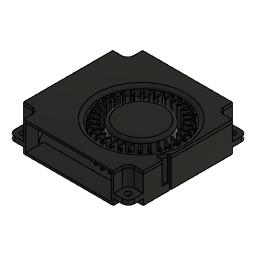
Fan centrifugal 40x40x10 v9 (Autodesk Fusion 360 design; units mm, degrees)
Autodesk Fusion 360 part; units mm, degrees
note: some values were not read from the file. Set by a fixed rule: which face or edge a step refers to; which sketch regions a step uses.
(part 1 of 2)
sketch "Sketch1" plane through (0, 0, 0) normal (0, 0, 1) x (1, 0, 0) in component "base"
  line L0 (18, 19.9) -> (-18, 19.9)
  line L1 (-18, -19.9) -> (18, -19.9)
  arc A0 (-20, -17.9) -> (-18, -19.9) centre (-18, -17.9) ccw
  line L2 (-15, -19.9) -> (-15, -16.9)
  line L3 (15, -16.9) -> (15, -19.9)
  line L4 (-20, 17.9) -> (-20, -17.9)
  arc A1 (-18, 19.9) -> (-20, 17.9) centre (-18, 17.9) ccw
  line L5 (-17, -14.9) -> (-20, -14.9)
  arc A2 (18.3387, -8.5746) -> (17.9789, -8) centre (18.3387, -8.1746) cw
  arc A3 (20, 17.9) -> (18, 19.9) centre (18, 17.9) ccw
  arc A4 (17, -14.9) -> (15, -16.9) centre (17, -16.9) ccw
  line L6 (17.9789, -8) -> (19.0465, -5.8)
  line L7 (19.4063, -5.5746) -> (20, -5.5746)
  arc A5 (19.0465, -5.8) -> (19.4063, -5.5746) centre (19.4063, -5.9746) cw
  line L8 (20, -17.9) -> (20, 17.9)
  circle A6 centre (17.5, -17.5) radius 1
  circle A7 centre (17.5, 17.5) radius 1
  line L9 (19.5, -5.5746) -> (19.5, -8.5746)
  line L10 (20, -14.9) -> (17, -14.9)
  circle A8 centre (-17.5, -17.5) radius 1
  arc A9 (-15, -16.9) -> (-17, -14.9) centre (-17, -16.9) ccw
  circle A10 centre (-17.5, 17.5) radius 1
  arc A11 (18, -19.9) -> (20, -17.9) centre (18, -17.9) ccw
  line L11 (20, -8.5746) -> (18.3387, -8.5746)
  line L12 (18, 17.9) -> (-18, -17.9) construction
  line L13 (-18, 17.9) -> (18, -17.9) construction
  line L14 (0, 0) -> (0, 8.903) construction
  line L15 (17.9789, -8) -> (17.7, -8.5746) construction
  line L16 (18.3387, -8.5746) -> (17.7, -8.5746) construction
  line L17 (0, 0) -> (8.2242, 0) construction
  line L18 (-15, 19.9) -> (-15, 16.9)
  arc A12 (-17, 14.9) -> (-15, 16.9) centre (-17, 16.9) ccw
  line L19 (-17, 14.9) -> (-20, 14.9)
  line L20 (15, 19.9) -> (15, 16.9)
  arc A13 (15, 16.9) -> (17, 14.9) centre (17, 16.9) ccw
  line L21 (17, 14.9) -> (20, 14.9)
  line L22 (14, -19.9) -> (14, -10.4)
  line L23 (-14, -19.9) -> (-14, -15.9)
  line L24 (19.5, 8.2159) -> (19.5, -2.135) construction
  line L25 (-2.9229, 19.25) -> (4.8128, 19.25) construction
  arc A14 (14, -10.4) -> (19.5, 1.2082) centre (4.5, 1.2082) ccw
  arc A15 (19.5, 1.2082) -> (1.4582, 19.25) centre (1.4582, 1.2082) ccw
  arc A16 (1.4582, 19.25) -> (-19.5, -1.7082) centre (1.4582, -1.7082) ccw
  line L26 (-19.5, 5.9603) -> (-19.5, -4.1012) construction
  arc A17 (-19.5, -1.7082) -> (-14, -15.9) centre (1.5598, -1.7082) ccw
  line L27 (19.5, -6.0746) -> (20, -6.0746)
  circle A18 centre (0, 0) radius 12.5
  circle A19 centre (4.5, -0.1) radius 3
  line L28 (4.5, -0.1) -> (18.5127, -6.9) construction
  line L29 (18.1641, -8.5345) -> (12.3384, -5.7074)
  line L30 (19.5, -5.5746) -> (13.7556, -2.787)
  line L31 (13.92, -2.4482) -> (12.1736, -6.0469)
  arc A20 (10.8374, -6.51) -> (12.1736, -6.0469) centre (11.274, -5.6103) ccw
  line L32 (10.8374, -6.51) -> (7.6886, -4.9819)
  arc A21 (7.2255, -3.6457) -> (7.6886, -4.9819) centre (8.1251, -4.0822) ccw
  line L33 (7.2255, -3.6457) -> (8.9718, -0.047)
  arc A22 (10.3081, 0.4161) -> (8.9718, -0.047) centre (9.8715, -0.4836) ccw
  line L34 (10.3081, 0.4161) -> (13.4569, -1.112)
  arc A23 (13.92, -2.4482) -> (13.4569, -1.112) centre (13.0203, -2.0116) ccw
  dimension "d2" = 40
  dimension "d3" = 39.8
  dimension "d10" = 2
  dimension "d12" = 2
  dimension "d13" = 5
  dimension "d18" = 3
  dimension "d21" = 35
  dimension "d22" = 35
  dimension "d23" = 0.5
  dimension "d26" = 2.3
  dimension "d27" = 5
  dimension "d28" = 5
  dimension "d29" = 2
  dimension "d30" = 0.4
  dimension "d31" = 9.5
  dimension "d32" = 28
  dimension "d33" = 0.5
  dimension "d34" = 0.65
  dimension "d35" = 0.5
  dimension "d36" = 4
  dimension "d37" = 15
  dimension "d38" = 0.5
  dimension "d97" = 25
  dimension "d98" = 6
  dimension "d99" = 15.5
  dimension "d100" = 20
  dimension "d101" = 8
  dimension "d102" = 1
  dimension "d103" = 6
  dimension "d104" = 9.5
  dimension "d105" = 5.5
  constraint coincident L9.start L7
  constraint tangent L0 A1
  constraint tangent L4 A1
  constraint tangent A3 L8
  constraint tangent L0 A3
  constraint tangent L5 A9
  constraint tangent A0 L4
  constraint tangent L8 A11
  constraint tangent A4 L10
  constraint tangent A2 L11
  constraint tangent A2 L6
  constraint tangent L7 A5
  constraint tangent L6 A5
  constraint coincident A3.centre L12.start
  constraint coincident A0.centre L12.end
  constraint coincident A1.centre L13.start
  constraint coincident A11.centre L13.end
  constraint midpoint L12 L14.start
  constraint equal A7 A10
  constraint equal A6 A7
  constraint equal A6 A8
  constraint equal A1 A3
  constraint equal A3 A11
  constraint equal A0 A11
  constraint equal A4 A9
  constraint vertical L4
  constraint vertical L8
  constraint horizontal L0
  constraint horizontal L1
  constraint tangent L1 A0
  constraint tangent L1 A11
  constraint coincident L9.end L11
  constraint horizontal L11
  constraint vertical L9
  constraint horizontal L7
  constraint horizontal L10
  constraint vertical L3
  constraint vertical L2
  constraint horizontal L5
  constraint tangent L2 A9
  constraint collinear L5 L10
  constraint coincident L14.start L17.start
  constraint parallel L6 L15
  constraint parallel L11 L16
  constraint equal A2 A5
  constraint tangent L3 A4
  constraint vertical L14
  constraint horizontal L17
  constraint symmetric A6.centre A7.centre L17
  constraint symmetric A8.centre A10.centre L17
  constraint symmetric A6.centre A8.centre L14
  constraint coincident L10.start L8
  constraint coincident L3.start A4.end
  constraint coincident L3.end L1
  constraint coincident L5.end L4
  constraint coincident L2.start L1
  constraint coincident L2.end A9.start
  constraint symmetric L3.end L2.start L14
  constraint coincident L0 L18.start
  constraint tangent L18 A12
  constraint coincident L4 L19.end
  constraint tangent A12 L19
  constraint coincident L0 L20.start
  constraint tangent L20 A13
  constraint coincident L8 L21.end
  constraint tangent A13 L21
  constraint vertical L18
  constraint horizontal L19
  constraint vertical L20
  constraint horizontal L21
  constraint collinear L19 L21
  constraint collinear L2 L18
  constraint collinear L3 L20
  constraint equal A9 A12
  constraint equal A9 A13
  constraint coincident L7.end L8
  constraint coincident L8 L11.start
  constraint coincident L1 L22.start
  constraint perpendicular L1 L22
  constraint coincident L1 L23.start
  constraint perpendicular L1 L23
  constraint vertical L24
  constraint symmetric L14 L22.start L23.start
  constraint horizontal L25
  constraint tangent L24 A14
  constraint coincident L24 A14.end
  constraint tangent L25 A15
  constraint coincident L25 A15.end
  constraint tangent L24 A15
  constraint tangent L25 A16
  constraint vertical L26
  constraint tangent A16 L26
  constraint coincident A16.end L26
  constraint tangent L26 A17
  constraint coincident L9 L27.start
  constraint coincident L8 L27.end
  constraint perpendicular L8 L27
  constraint coincident A19.centre L28.start
  constraint midpoint L6 L28.end
  constraint perpendicular L6 L28
  constraint coincident A2 L29.start
  constraint tangent A2 L29
  constraint parallel L28 L29
  constraint parallel L28 L30
  constraint perpendicular L28 L31
  constraint tangent L31 A20
  constraint tangent A20 L32
  constraint tangent L32 A21
  constraint tangent A21 L33
  constraint tangent L33 A22
  constraint tangent A22 L34
  constraint tangent L34 A23
  constraint tangent L31 A23
  constraint perpendicular L28 L33
  constraint parallel L28 L34
  constraint parallel L28 L32
  constraint equal A22 A23
  constraint equal A21 A22
  constraint equal A20 A21
  constraint symmetric L28 A20.start L34.end
  constraint coincident L30.end L31
  constraint coincident L29.end L31
  measures "d2" distance of L4 L8
  measures "d3" distance of L0 L1
  measures "d10" radius of A1
  measures "d12" diameter of A10
  measures "d13" distance of L1 L5
  measures "d18" distance of L7 L11
  measures "d21" distance of A6.centre A7.centre
  measures "d22" distance of A7.centre A10.centre
  measures "d23" distance of L8 L9
  measures "d26" distance of L8 L15.end
  measures "d27" distance of L2 L4
  measures "d28" distance of L0 L19
  measures "d29" radius of A12
  measures "d30" radius of A2
  measures "d31" distance of L22.start L22.end
  measures "d32" distance of L22 L23
  measures "d33" distance of L8 L24
  measures "d34" distance of L0 L25
  measures "d35" distance of L4 L26
  measures "d36" distance of L23.start L23.end
  measures "d37" radius of A14
  measures "d38" distance of L7 L27
  measures "d97" diameter of A18
  measures "d98" diameter of A19
  measures "d99" distance of L8 A19.centre
  measures "d100" distance of L0 A19.centre
  measures "d101" distance of L10 L28.end
  measures "d102" radius of A21
  measures "d103" distance of L32 L34
  measures "d104" distance of A19.centre L31
  measures "d105" distance of L31 L33
extrude "Extrude1" add sketch "Sketch1" along normal blind 9 contours L0 L1 L2 L4 L5 L7 L8 A9 L18 A12 L19 L20 A13 L21 L23 A14 A15 A16 A17 L30 | A2 L6 L7 A5 A14 L29 L30 | L1 L22 L23 A14 A15 A16 A17 A18 L29 L30 L31 A20 L32 L34 A23 | A14 L29 L30 L31 | L1 L3 A2 A4 L8 L10 L11 L22 A14 L29 | A18 L31 A20 L32 L34 A23 | A18 L32 A21 L33 A22 L34 | A18 L32 A21 L33 A22 L34 | A19 makes body 1 in component "base"
extrude "Extrude2" add sketch "Sketch1" along normal blind 1.5 from surface at 2 contours L0 A3 L8 L20 A13 L21 | L0 L4 A1 L18 A12 L19 | L1 A0 L2 L4 L5 A9 | L1 L3 A4 L8 L10 A11 bodies 1 in component "base"
extrude "Extrude3" cut sketch "Sketch1" along normal through all from surface at 1 contours L1 L22 L23 A14 A15 A16 A17 A18 L29 L30 L31 A20 L32 L34 A23 | A14 L29 L30 L31 | A18 L31 A20 L32 L34 A23 | A18 L32 A21 L33 A22 L34 | A18 L32 A21 L33 A22 L34 | A19 bodies 1 in component "base"
shell "Shell1" thickness 0.75 removed faces 1 at (-4.4672, -2.6667, 0) on bodies 1 in component "base"
sketch "Sketch2" plane through (0, 0, 8.25) normal (0, 0, -1) x (1, 0, 0) in component "base"
  line L0 (19.25, 4.3145) -> (19.25, 4.8353)
  arc A0 (19.25, 4.3145) -> (19.0211, 4.8911) centre (4.5, -1.2082) ccw
  arc A1 (18.3387, 9.3246) -> (17.19, 8.1206) centre (18.3387, 8.1746) ccw
  line L1 (18.3387, 9.3246) -> (19.25, 9.3246)
  line L2 (19.25, 9.3246) -> (19.25, 14.15)
  line L3 (19.25, 14.15) -> (17, 14.15)
  arc A2 (14.75, 15.3189) -> (17, 14.15) centre (17, 16.9) ccw
  line L4 (14.75, 15.3189) -> (14.75, 10.7501)
  arc A3 (17.19, 8.1206) -> (14.75, 10.7501) centre (4.5, -1.2082) ccw
  arc A4 (-17, 14.15) -> (-16.2874, 14.2439) centre (-17, 16.9) ccw
  line L5 (-17, 14.15) -> (-19.25, 14.15)
  line L6 (-19.25, 14.15) -> (-19.25, 8.2366)
  arc A5 (-16.2874, 14.2439) -> (-19.25, 8.2366) centre (1.5598, 1.7082) ccw
  line L7 (-19.25, -4.8046) -> (-19.25, -14.15)
  line L8 (-19.25, -14.15) -> (-17, -14.15)
  arc A6 (-14.25, -16.9) -> (-17, -14.15) centre (-17, -16.9) ccw
  line L9 (-14.25, -16.9) -> (-14.25, -19.15)
  line L10 (-14.25, -19.15) -> (-4.5569, -19.15)
  arc A7 (-19.25, -4.8046) -> (-4.5569, -19.15) centre (1.4582, 1.7082) ccw
  line L11 (7.046, -19.15) -> (14.25, -19.15)
  line L12 (14.25, -19.15) -> (14.25, -16.9)
  arc A8 (17, -14.15) -> (14.25, -16.9) centre (17, -16.9) ccw
  line L13 (17, -14.15) -> (19.25, -14.15)
  line L14 (19.25, -14.15) -> (19.25, -7.2566)
  arc A9 (7.046, -19.15) -> (19.25, -7.2566) centre (1.4582, -1.2082) ccw
  arc A10 (19.0211, 4.8911) -> (19.25, 4.8353) centre (19.4063, 5.9746) ccw
  line L15 (18.3387, 9.3246) -> (16.2099, 9.3246)
  arc A11 (14.6087, -15.5421) -> (14.0867, -15.1241) centre (14.3142, -15.3749) ccw
  circle A12 centre (17.5, -17.5) radius 1
  line L16 (17.5, -17.5) -> (0, 0) construction
  arc A13 (15.1387, -14.0914) -> (15.5349, -14.5728) centre (15.3674, -14.3068) ccw
  dimension "d115" = 1.5
  dimension "d116" = 0.75
  constraint coincident A1.start L1.start
  constraint coincident A3 L15.end
  constraint tangent A1 L15
  constraint coincident A8 A11.start
  constraint coincident A9 A11.end
  constraint coincident A12.centre L16.start
  constraint coincident L16.end origin
  constraint tangent A8 A11
  constraint tangent A9 A11
  constraint coincident A8 A13.end
  constraint coincident A9 A13.start
  constraint tangent A9 A13
  constraint tangent A8 A13
  measures "d115" distance of A11.centre A13.centre
  measures "d116" distance of A11.centre L16
sketch "Sketch4" plane through (0, 0, 0.25) normal (0, 0, -1) x (1, 0, 0) in component "base"
  line L0 (-4.5569, -19.15) -> (7.046, -19.15)
  arc A0 (7.046, -19.15) -> (19.25, -7.2566) centre (1.4582, -1.2082) ccw
  line L1 (19.25, -7.2566) -> (19.25, 4.3145)
  arc A1 (19.25, 4.3145) -> (19.0211, 4.8911) centre (4.5, -1.2082) ccw
  arc A2 (18.3717, 5.4726) -> (19.0211, 4.8911) centre (19.4063, 5.9746) ccw
  line L2 (18.3717, 5.4726) -> (17.3041, 7.6726)
  arc A3 (17.19, 8.1206) -> (17.3041, 7.6726) centre (18.3387, 8.1746) ccw
  arc A4 (17.19, 8.1206) -> (14.75, 10.7501) centre (4.5, -1.2082) ccw
  line L3 (14.75, 10.7501) -> (14.75, 15.3189)
  arc A5 (14.25, 16.9) -> (14.75, 15.3189) centre (17, 16.9) ccw
  line L4 (14.25, 16.9) -> (14.25, 19.15)
  line L5 (14.25, 19.15) -> (-14.25, 19.15)
  line L6 (-14.25, 19.15) -> (-14.25, 16.9)
  arc A6 (-16.2874, 14.2439) -> (-14.25, 16.9) centre (-17, 16.9) ccw
  arc A7 (-16.2874, 14.2439) -> (-19.25, 8.2366) centre (1.5598, 1.7082) ccw
  line L7 (-19.25, 8.2366) -> (-19.25, -4.8046)
  arc A8 (-19.25, -4.8046) -> (-4.5569, -19.15) centre (1.4582, 1.7082) ccw
extrude "Extrude10" add sketch "Sketch4" along normal up to surface (0.25 mm away) bodies 1 in component "base"
extrude "Extrude4" add sketch "Sketch2" along normal up to surface (8.25 mm away) contours L0 A0 A10 | A1 A3 L15 | A8 A9 A11 A13 bodies 1 in component "base"
extrude "Extrude5" add sketch "Sketch2" along normal blind 2.25 contours L1 L2 L3 A2 L4 A3 L15 | A1 A3 L15 | A4 L5 L6 A5 | L7 L8 A6 L9 L10 A7 | L11 L12 A8 A9 A11 | A8 A9 A11 A13 | A8 L13 L14 A9 A13 bodies 1 in component "base"
sketch "Sketch3" plane through (0, 0, 9) normal (0, 0, 1) x (-1, 0, 0) in component "base"
  arc A0 (19.5, 1.7082) -> (14, 15.9) centre (-1.5598, 1.7082) ccw
  arc A1 (-1.4582, -19.25) -> (19.5, 1.7082) centre (-1.4582, 1.7082) ccw
  arc A2 (-19.5, -1.2082) -> (-1.4582, -19.25) centre (-1.4582, -1.2082) ccw
  arc A3 (-14, 10.4) -> (-19.5, -1.2082) centre (-4.5, -1.2082) ccw
  line L0 (-14, 10.4) -> (-14, 19.9)
  line L1 (-14, 19.9) -> (-15, 19.9)
  line L2 (-15, 19.9) -> (-15, 16.9)
  arc A4 (-17, 14.9) -> (-15, 16.9) centre (-17, 16.9) ccw
  line L3 (-17, 14.9) -> (-20, 14.9)
  line L4 (-20, 14.9) -> (-20, 8.5746)
  line L5 (-20, 8.5746) -> (-18.3387, 8.5746)
  arc A5 (-17.9789, 8) -> (-18.3387, 8.5746) centre (-18.3387, 8.1746) ccw
  line L6 (-17.9789, 8) -> (-19.0465, 5.8)
  arc A6 (-19.4063, 5.5746) -> (-19.0465, 5.8) centre (-19.4063, 5.9746) ccw
  line L7 (-19.4063, 5.5746) -> (-20, 5.5746)
  line L8 (-20, 5.5746) -> (-20, -14.9)
  line L9 (-20, -14.9) -> (-17, -14.9)
  arc A7 (-15, -16.9) -> (-17, -14.9) centre (-17, -16.9) ccw
  line L10 (-15, -16.9) -> (-15, -19.9)
  line L11 (-15, -19.9) -> (15, -19.9)
  line L12 (15, -19.9) -> (15, -16.9)
  arc A8 (17, -14.9) -> (15, -16.9) centre (17, -16.9) ccw
  line L13 (17, -14.9) -> (20, -14.9)
  line L14 (20, -14.9) -> (20, 14.9)
  line L15 (20, 14.9) -> (17, 14.9)
  arc A9 (15, 16.9) -> (17, 14.9) centre (17, 16.9) ccw
  line L16 (15, 16.9) -> (15, 19.9)
  line L17 (15, 19.9) -> (14, 19.9)
  circle A10 centre (-14.5, 14.9) radius 0.4
  line L18 (-14.5, 13.85) -> (-14.5, 14.15)
  arc A11 (-14.5, 14.15) -> (-14.75, 14.4) centre (-14.75, 14.15) ccw
  line L19 (-14.75, 14.4) -> (-18.5, 14.4)
  arc A12 (-18.5, 14.4) -> (-19.5, 13.4) centre (-18.5, 13.4) ccw
  line L20 (-19.5, 13.4) -> (-19.5, 10.9746)
  arc A13 (-19.5, 10.9746) -> (-18.5, 9.9746) centre (-18.5, 10.9746) ccw
  line L21 (-18.5, 9.9746) -> (-16.1768, 9.9746)
  arc A14 (-16.1768, 9.9746) -> (-15.9419, 10.1391) centre (-16.1768, 10.2246) ccw
  line L22 (-15.9419, 10.1391) -> (-15.8327, 10.4391)
  arc A15 (-15.8327, 10.4391) -> (-16.0676, 10.7746) centre (-16.0676, 10.5246) ccw
  line L23 (-16.0676, 10.7746) -> (-18.35, 10.7746)
  arc A16 (-18.7, 11.1246) -> (-18.35, 10.7746) centre (-18.35, 11.1246) ccw
  line L24 (-18.7, 11.1246) -> (-18.7, 13.25)
  arc A17 (-18.35, 13.6) -> (-18.7, 13.25) centre (-18.35, 13.25) ccw
  line L25 (-18.35, 13.6) -> (-14.75, 13.6)
  arc A18 (-14.75, 13.6) -> (-14.5, 13.85) centre (-14.75, 13.85) ccw
  line L26 (-20, 8.9746) -> (-18.3387, 8.9746)
  arc A19 (-17.619, 7.8254) -> (-18.3387, 8.9746) centre (-18.3387, 8.1746) ccw
  line L27 (-17.619, 7.8254) -> (-18.6866, 5.6254)
  arc A20 (-19.4063, 5.1746) -> (-18.6866, 5.6254) centre (-19.4063, 5.9746) ccw
  line L28 (-19.4063, 5.1746) -> (-20, 5.1746)
  line L29 (-9.25, -19.4) -> (-13, -19.4)
  arc A21 (-14.5, -17.9) -> (-13, -19.4) centre (-13, -17.9) ccw
  line L30 (-14.5, -17.9) -> (-14.5, -16.9)
  arc A22 (-14.5, -16.9) -> (-17, -14.4) centre (-17, -16.9) ccw
  line L31 (-17, -14.4) -> (-18, -14.4)
  arc A23 (-19.5, -12.9) -> (-18, -14.4) centre (-18, -12.9) ccw
  line L32 (-19.5, -12.9) -> (-19.5, -9.15)
  line L33 (-9.25, -18.6) -> (-13, -18.6)
  arc A24 (-13.7, -17.9) -> (-13, -18.6) centre (-13, -17.9) ccw
  line L34 (-13.7, -17.9) -> (-13.7, -16.9)
  arc A25 (-13.7, -16.9) -> (-17, -13.6) centre (-17, -16.9) ccw
  line L35 (-17, -13.6) -> (-18, -13.6)
  arc A26 (-18.7, -12.9) -> (-18, -13.6) centre (-18, -12.9) ccw
  line L36 (-18.7, -12.9) -> (-18.7, -9.15)
  arc A27 (-9.25, -19.4) -> (-9, -19.15) centre (-9.25, -19.15) ccw
  line L37 (-9, -19.15) -> (-9, -18.85)
  arc A28 (-9, -18.85) -> (-9.25, -18.6) centre (-9.25, -18.85) ccw
  arc A29 (-18.7, -9.15) -> (-18.95, -8.9) centre (-18.95, -9.15) ccw
  line L38 (-18.95, -8.9) -> (-19.25, -8.9)
  arc A30 (-19.25, -8.9) -> (-19.5, -9.15) centre (-19.25, -9.15) ccw
  circle A31 centre (-19, -7.9) radius 0.5
  line L39 (7.25, -19.4) -> (13, -19.4)
  arc A32 (13, -19.4) -> (14.5, -17.9) centre (13, -17.9) ccw
  line L40 (14.5, -17.9) -> (14.5, -16.9)
  arc A33 (17, -14.4) -> (14.5, -16.9) centre (17, -16.9) ccw
  line L41 (17, -14.4) -> (18, -14.4)
  arc A34 (18, -14.4) -> (19.5, -12.9) centre (18, -12.9) ccw
  line L42 (19.5, -12.9) -> (19.5, -6.65)
  line L43 (7.25, -18.6) -> (13, -18.6)
  arc A35 (13, -18.6) -> (13.7, -17.9) centre (13, -17.9) ccw
  line L44 (13.7, -17.9) -> (13.7, -16.9)
  arc A36 (17, -13.6) -> (13.7, -16.9) centre (17, -16.9) ccw
  line L45 (17, -13.6) -> (18, -13.6)
  arc A37 (18, -13.6) -> (18.7, -12.9) centre (18, -12.9) ccw
  line L46 (18.7, -12.9) -> (18.7, -6.65)
  arc A38 (7, -19.15) -> (7.25, -19.4) centre (7.25, -19.15) ccw
  line L47 (7, -19.15) -> (7, -18.85)
  arc A39 (7.25, -18.6) -> (7, -18.85) centre (7.25, -18.85) ccw
  arc A40 (19.5, -6.65) -> (19.25, -6.4) centre (19.25, -6.65) ccw
  line L48 (19.25, -6.4) -> (18.95, -6.4)
  arc A41 (18.95, -6.4) -> (18.7, -6.65) centre (18.95, -6.65) ccw
  circle A42 centre (19, -5.4) radius 0.5
  line L49 (19.5, 9.15) -> (19.5, 13.4)
  arc A43 (19.5, 13.4) -> (18.5, 14.4) centre (18.5, 13.4) ccw
  line L50 (18.5, 14.4) -> (16.75, 14.4)
  line L51 (18.7, 9.15) -> (18.7, 13.4)
  arc A44 (18.7, 13.4) -> (18.5, 13.6) centre (18.5, 13.4) ccw
  line L52 (18.5, 13.6) -> (16.75, 13.6)
  arc A45 (16.75, 14.4) -> (16.5, 14.15) centre (16.75, 14.15) ccw
  line L53 (16.5, 14.15) -> (16.5, 13.85)
  arc A46 (16.5, 13.85) -> (16.75, 13.6) centre (16.75, 13.85) ccw
  arc A47 (18.7, 9.15) -> (18.95, 8.9) centre (18.95, 9.15) ccw
  line L54 (18.95, 8.9) -> (19.25, 8.9)
  arc A48 (19.25, 8.9) -> (19.5, 9.15) centre (19.25, 9.15) ccw
  line L55 (14, 19.9) -> (14, 15.9)
  dimension "d53" = 110
  dimension "d54" = 0.8
  dimension "d55" = 0.5
  dimension "d56" = -0.4
  dimension "d57" = 1
  dimension "d58" = 0.8
  dimension "d59" = 0.8
  dimension "d60" = 0.5
  dimension "d61" = 0.25
  dimension "d62" = 0.5
  dimension "d63" = 5
  dimension "d64" = 5.5
  dimension "d65" = 0.8
  dimension "d66" = 0.5
  dimension "d67" = 0.5
  dimension "d68" = 0.5
  dimension "d70" = 1.5
  dimension "d71" = 0.8
  dimension "d72" = 1
  dimension "d73" = 0.35
  dimension "d76" = 1
  dimension "d77" = 1
  dimension "d79" = -0.8
  dimension "d80" = 0.5
  dimension "d81" = 0.5
  dimension "d82" = 0.5
  dimension "d83" = 8.5
  dimension "d84" = 8
  dimension "d85" = 1
  dimension "d86" = 1
  dimension "d87" = 9.5
  dimension "d88" = 7
  dimension "d89" = 6
  dimension "d90" = 6
  dimension "d91" = 1
  dimension "d92" = -0.8
  dimension "d93" = 0.5
  dimension "d94" = 0.5
  dimension "d95" = 3.5
  dimension "d96" = 6
  constraint vertical L18
  constraint tangent L18 A11
  constraint horizontal L19
  constraint tangent L19 A12
  constraint perpendicular L19 L20
  constraint tangent L20 A13
  constraint tangent A13 L21
  constraint horizontal L21
  constraint tangent L21 A14
  constraint tangent A14 L22
  constraint tangent L22 A15
  constraint tangent L23 A16
  constraint tangent L24 A17
  constraint tangent L25 A18
  constraint parallel L21 L23
  constraint parallel L20 L24
  constraint parallel L19 L25
  constraint tangent L18 A18
  constraint tangent A11 L19
  constraint tangent A12 L20
  constraint tangent A17 L25
  constraint tangent A16 L24
  constraint tangent A15 L23
  constraint equal A14 A15
  constraint equal A11 A18
  constraint tangent A14 L27
  constraint horizontal L29
  constraint tangent L29 A21
  constraint perpendicular L29 L30
  constraint tangent L30 A22
  constraint perpendicular L30 L31
  constraint tangent L31 A23
  constraint perpendicular L31 L32
  constraint tangent A21 L30
  constraint tangent A23 L32
  constraint concentric A7 A22
  constraint tangent A22 L31
  constraint equal A21 A23
  constraint equal A15 A18
  constraint equal A12 A13
  constraint equal A16 A17
  constraint tangent L29 A27
  constraint perpendicular L29 L37
  constraint tangent L37 A28
  constraint tangent L36 A29
  constraint perpendicular L36 L38
  constraint tangent L38 A30
  constraint tangent L32 A30
  constraint tangent A29 L38
  constraint tangent A27 L37
  constraint tangent L33 A28
  constraint equal A29 A30
  constraint equal A27 A29
  constraint equal A27 A28
  constraint equal A18 A28
  constraint tangent L39 A32
  constraint tangent A32 L40
  constraint tangent L40 A33
  constraint tangent L41 A34
  constraint vertical L42
  constraint tangent A33 L41
  constraint horizontal L41
  constraint horizontal L39
  constraint vertical L40
  constraint tangent A34 L42
  constraint concentric A8 A33
  constraint equal A32 A34
  constraint equal A21 A32
  constraint tangent L39 A38
  constraint perpendicular L39 L47
  constraint tangent L47 A39
  constraint tangent A38 L47
  constraint tangent L43 A39
  constraint tangent L42 A40
  constraint perpendicular L42 L48
  constraint tangent L48 A41
  constraint tangent L46 A41
  constraint tangent A40 L48
  constraint equal A38 A39
  constraint equal A39 A40
  constraint equal A40 A41
  constraint equal A18 A41
  constraint vertical L49
  constraint tangent L49 A43
  constraint tangent A43 L50
  constraint horizontal L50
  constraint tangent L50 A45
  constraint perpendicular L50 L53
  constraint tangent L53 A46
  constraint tangent L51 A47
  constraint perpendicular L51 L54
  constraint tangent L54 A48
  constraint tangent L49 A48
  constraint tangent A47 L54
  constraint tangent L52 A46
  constraint tangent A45 L53
  constraint equal A45 A46
  constraint equal A46 A47
  constraint equal A47 A48
  constraint equal A18 A47
  measures "d53" angle of L21 L22
  measures "d54" distance of L20 L24
  measures "d55" distance of L4 L20
  measures "d57" distance of L21 L26
  measures "d58" distance of L19 L25
  measures "d59" distance of L21 L23
  measures "d60" distance of L3 L19
  measures "d61" radius of A18
  measures "d62" distance of L0 L18
  measures "d63" distance of L1 A10.centre
  measures "d64" distance of L4 A10.centre
  measures "d65" diameter of A10
  measures "d66" distance of A7 A22
  measures "d67" distance of L11 L29
  measures "d68" distance of L8 L32
  measures "d70" radius of A21
  measures "d72" radius of A13
  measures "d73" radius of A16
  measures "d76" distance of L8 A31.centre
  measures "d77" diameter of A31
  measures "d80" distance of L11 L39
  measures "d81" distance of L14 L42
  measures "d82" distance of A8 A33
  measures "d83" distance of L13 L48
  measures "d84" distance of L12 L47
  measures "d85" diameter of A42
  measures "d86" distance of L14 A42.centre
  measures "d87" distance of L13 A42.centre
  measures "d88" distance of L9 A31.centre
  measures "d89" distance of L9 L38
  measures "d90" distance of L10 L37
  measures "d91" radius of A43
  measures "d93" distance of L14 L49
  measures "d94" distance of L15 L50
  measures "d95" distance of L14 L53
  measures "d96" distance of L15 L54
extrude "Extrude6" cut sketch "Sketch1" along normal blind 0.25 contours A18 L32 A21 L33 A22 L34 | A18 L32 A21 L33 A22 L34 | A19 bodies 1 in component "base"
extrude "Extrude7" cut sketch "Sketch1" along normal blind 0.75 contours A2 L6 L7 A5 A14 L29 L30 | A14 L29 L30 L31 bodies 1 in component "base"
extrude "Extrude8" cut sketch "Sketch1" along normal through all contours A18 L31 A20 L32 L34 A23 | A18 L32 A21 L33 A22 L34 picked at (9.3839, -2.4486) bodies 1 in component "base"
extrude "Extrude9" add sketch "Sketch1" along normal blind 2.4 contours L8 L9 L11 L27 bodies 1 in component "base"
extrude "Extrude11" cut sketch "Sketch3" against normal blind 1.5 contours A10 | L18 A11 L19 A12 L20 A13 L21 A14 L22 A15 L23 A16 L24 A17 L25 A18 | L29 A21 L30 A22 L31 A23 L32 L33 A24 L34 A25 L35 A26 L36 A27 L37 A28 A29 L38 A30 | A31 | L39 A32 L40 A33 L41 A34 L42 L43 A35 L44 A36 L45 A37 L46 A38 L47 A39 A40 L48 A41 | A42 | L49 A43 L50 L51 A44 L52 A45 L53 A46 A47 L54 A48 bodies 1 in component "base"
sketch "Sketch1 (2)" plane through (0, 0, 9) normal (0, 0, 1) x (-1, 0, 0) in component "lid"
  circle A0 centre (19, -5.4) radius 0.5
  arc A1 (18, -14.4) -> (19.5, -12.9) centre (18, -12.9) ccw
  line L0 (18, -14.4) -> (17, -14.4)
  arc A2 (17, -14.4) -> (14.5, -16.9) centre (17, -16.9) ccw
  line L1 (14.5, -16.9) -> (14.5, -17.9)
  arc A3 (13, -19.4) -> (14.5, -17.9) centre (13, -17.9) ccw
  line L2 (13, -19.4) -> (7.25, -19.4)
  arc A4 (7, -19.15) -> (7.25, -19.4) centre (7.25, -19.15) ccw
  line L3 (7, -19.15) -> (7, -18.85)
  arc A5 (7.25, -18.6) -> (7, -18.85) centre (7.25, -18.85) ccw
  line L4 (7.25, -18.6) -> (13, -18.6)
  arc A6 (13, -18.6) -> (13.7, -17.9) centre (13, -17.9) ccw
  line L5 (13.7, -17.9) -> (13.7, -16.9)
  arc A7 (17, -13.6) -> (13.7, -16.9) centre (17, -16.9) ccw
  line L6 (17, -13.6) -> (18, -13.6)
  arc A8 (18, -13.6) -> (18.7, -12.9) centre (18, -12.9) ccw
  line L7 (18.7, -12.9) -> (18.7, -6.65)
  arc A9 (18.95, -6.4) -> (18.7, -6.65) centre (18.95, -6.65) ccw
  line L8 (18.95, -6.4) -> (19.25, -6.4)
  arc A10 (19.5, -6.65) -> (19.25, -6.4) centre (19.25, -6.65) ccw
  line L9 (19.5, -6.65) -> (19.5, -12.9)
  line L10 (19.25, 8.9) -> (18.95, 8.9)
  arc A11 (18.7, 9.15) -> (18.95, 8.9) centre (18.95, 9.15) ccw
  line L11 (18.7, 9.15) -> (18.7, 13.4)
  arc A12 (18.7, 13.4) -> (18.5, 13.6) centre (18.5, 13.4) ccw
  line L12 (18.5, 13.6) -> (16.75, 13.6)
  arc A13 (16.5, 13.85) -> (16.75, 13.6) centre (16.75, 13.85) ccw
  line L13 (16.5, 13.85) -> (16.5, 14.15)
  arc A14 (16.75, 14.4) -> (16.5, 14.15) centre (16.75, 14.15) ccw
  line L14 (16.75, 14.4) -> (18.5, 14.4)
  arc A15 (19.5, 13.4) -> (18.5, 14.4) centre (18.5, 13.4) ccw
  line L15 (19.5, 13.4) -> (19.5, 9.15)
  arc A16 (19.25, 8.9) -> (19.5, 9.15) centre (19.25, 9.15) ccw
  circle A17 centre (-19, -7.9) radius 0.5
  arc A18 (-18.7, -9.15) -> (-18.95, -8.9) centre (-18.95, -9.15) ccw
  line L16 (-18.7, -9.15) -> (-18.7, -12.9)
  arc A19 (-18.7, -12.9) -> (-18, -13.6) centre (-18, -12.9) ccw
  line L17 (-18, -13.6) -> (-17, -13.6)
  arc A20 (-13.7, -16.9) -> (-17, -13.6) centre (-17, -16.9) ccw
  line L18 (-13.7, -16.9) -> (-13.7, -17.9)
  arc A21 (-13.7, -17.9) -> (-13, -18.6) centre (-13, -17.9) ccw
  line L19 (-13, -18.6) -> (-9.25, -18.6)
  arc A22 (-9, -18.85) -> (-9.25, -18.6) centre (-9.25, -18.85) ccw
  line L20 (-9, -18.85) -> (-9, -19.15)
  arc A23 (-9.25, -19.4) -> (-9, -19.15) centre (-9.25, -19.15) ccw
  line L21 (-9.25, -19.4) -> (-13, -19.4)
  arc A24 (-14.5, -17.9) -> (-13, -19.4) centre (-13, -17.9) ccw
  line L22 (-14.5, -17.9) -> (-14.5, -16.9)
  arc A25 (-14.5, -16.9) -> (-17, -14.4) centre (-17, -16.9) ccw
  line L23 (-17, -14.4) -> (-18, -14.4)
  arc A26 (-19.5, -12.9) -> (-18, -14.4) centre (-18, -12.9) ccw
  line L24 (-19.5, -12.9) -> (-19.5, -9.15)
  arc A27 (-19.25, -8.9) -> (-19.5, -9.15) centre (-19.25, -9.15) ccw
  line L25 (-19.25, -8.9) -> (-18.95, -8.9)
  arc A28 (-14.75, 13.6) -> (-14.5, 13.85) centre (-14.75, 13.85) ccw
  line L26 (-14.75, 13.6) -> (-18.35, 13.6)
  arc A29 (-18.35, 13.6) -> (-18.7, 13.25) centre (-18.35, 13.25) ccw
  line L27 (-18.7, 13.25) -> (-18.7, 11.1246)
  arc A30 (-18.7, 11.1246) -> (-18.35, 10.7746) centre (-18.35, 11.1246) ccw
  line L28 (-18.35, 10.7746) -> (-16.0676, 10.7746)
  arc A31 (-15.8327, 10.4391) -> (-16.0676, 10.7746) centre (-16.0676, 10.5246) ccw
  line L29 (-15.8327, 10.4391) -> (-15.9419, 10.1391)
  arc A32 (-16.1768, 9.9746) -> (-15.9419, 10.1391) centre (-16.1768, 10.2246) ccw
  line L30 (-16.1768, 9.9746) -> (-18.5, 9.9746)
  arc A33 (-19.5, 10.9746) -> (-18.5, 9.9746) centre (-18.5, 10.9746) ccw
  line L31 (-19.5, 10.9746) -> (-19.5, 13.4)
  arc A34 (-18.5, 14.4) -> (-19.5, 13.4) centre (-18.5, 13.4) ccw
  line L32 (-18.5, 14.4) -> (-14.75, 14.4)
  arc A35 (-14.5, 14.15) -> (-14.75, 14.4) centre (-14.75, 14.15) ccw
  line L33 (-14.5, 14.15) -> (-14.5, 13.85)
  circle A36 centre (-14.5, 14.9) radius 0.4
  arc A37 (19.5, 1.7082) -> (14, 15.9) centre (-1.5598, 1.7082) ccw
  arc A38 (-1.4582, -19.25) -> (19.5, 1.7082) centre (-1.4582, 1.7082) ccw
  arc A39 (-19.5, -1.2082) -> (-1.4582, -19.25) centre (-1.4582, -1.2082) ccw
  arc A40 (-14, 10.4) -> (-19.5, -1.2082) centre (-4.5, -1.2082) ccw
  line L34 (-14, 10.4) -> (-14, 19.9)
  line L35 (-14, 19.9) -> (-15, 19.9)
  line L36 (-15, 19.9) -> (-15, 16.9)
  arc A41 (-17, 14.9) -> (-15, 16.9) centre (-17, 16.9) ccw
  line L37 (-17, 14.9) -> (-20, 14.9)
  line L38 (-20, 14.9) -> (-20, 8.5746)
  line L39 (-20, 8.5746) -> (-18.3387, 8.5746)
  arc A42 (-17.9789, 8) -> (-18.3387, 8.5746) centre (-18.3387, 8.1746) ccw
  line L40 (-17.9789, 8) -> (-19.0465, 5.8)
  arc A43 (-19.4063, 5.5746) -> (-19.0465, 5.8) centre (-19.4063, 5.9746) ccw
  line L41 (-19.4063, 5.5746) -> (-20, 5.5746)
  line L42 (-20, 5.5746) -> (-20, -14.9)
  line L43 (-20, -14.9) -> (-17, -14.9)
  arc A44 (-15, -16.9) -> (-17, -14.9) centre (-17, -16.9) ccw
  line L44 (-15, -16.9) -> (-15, -19.9)
  line L45 (-15, -19.9) -> (15, -19.9)
  line L46 (15, -19.9) -> (15, -16.9)
  arc A45 (17, -14.9) -> (15, -16.9) centre (17, -16.9) ccw
  line L47 (17, -14.9) -> (20, -14.9)
  line L48 (20, -14.9) -> (20, 14.9)
  line L49 (20, 14.9) -> (17, 14.9)
  arc A46 (15, 16.9) -> (17, 14.9) centre (17, 16.9) ccw
  line L50 (15, 16.9) -> (15, 19.9)
  line L51 (15, 19.9) -> (14, 19.9)
  line L52 (14, 19.9) -> (-14, 19.9)
  line L53 (14, 19.9) -> (14, 15.9)
  constraint coincident L51.end L52.start
  constraint coincident L34.end L35.start
extrude "Extrude1'" add sketch "Sketch1 (2)" along normal blind 1 separate body contours A0 | A1 L0 A2 L1 A3 L2 A4 L3 A5 L4 A6 L5 A7 L6 A8 L7 A9 L8 A10 L9 | L10 A11 L11 A12 L12 A13 L13 A14 L14 A15 L15 A16 | A17 | A18 L16 A19 L17 A20 L18 A21 L19 A22 L20 A23 L21 A24 L22 A25 L23 A26 L24 A27 L25 | A28 L26 A29 L27 A30 L28 A31 L29 A32 L30 A33 L31 A34 L32 A35 L33 | A36 | A37 A38 A39 A40 L34 L52 L53 | A37 A38 A39 A40 L34 L35 L36 A41 L37 L38 L39 A42 L40 A43 L41 L42 L43 A44 L44 L45 L46 A45 L47 L48 L49 A46 L50 L51 L53 makes body 2 in component "lid"
extrude "Extrude2'" add sketch "Sketch1 (2)" against normal blind 1.4 contours A0 | A1 L0 A2 L1 A3 L2 A4 L3 A5 L4 A6 L5 A7 L6 A8 L7 A9 L8 A10 L9 | L10 A11 L11 A12 L12 A13 L13 A14 L14 A15 L15 A16 | A17 | A18 L16 A19 L17 A20 L18 A21 L19 A22 L20 A23 L21 A24 L22 A25 L23 A26 L24 A27 L25 | A28 L26 A29 L27 A30 L28 A31 L29 A32 L30 A33 L31 A34 L32 A35 L33 | A36 bodies 2 in component "lid"
sketch "Sketch1 (3)" plane through (0, -19.9, 0) normal (0, -1, 0) x (1, 0, 0)
  line L0 (14, 9) -> (14, 1)
  line L1 (14, 1) -> (-14, 1)
  line L2 (-14, 1) -> (-14, 9)
  line L3 (-14, 9) -> (-15, 9)
  line L4 (-15, 9) -> (-15, 3.5)
  line L5 (-15, 3.5) -> (-18, 3.5)
  line L6 (-18, 3.5) -> (-18, 2)
  line L7 (-18, 2) -> (-15, 2)
  line L8 (-15, 2) -> (-15, 0)
  line L9 (-15, 0) -> (15, 0)
  line L10 (15, 0) -> (15, 2)
  line L11 (15, 2) -> (18, 2)
  line L12 (18, 2) -> (18, 3.5)
  line L13 (18, 3.5) -> (15, 3.5)
  line L14 (15, 3.5) -> (15, 9)
  line L15 (15, 9) -> (14, 9)
  line L16 (-14, 9) -> (14, 9)
  line L17 (-14.3, 9.3) -> (14.3, 9.3)
  line L18 (14.3, 9.3) -> (14.3, 0.7)
  line L19 (14.3, 0.7) -> (-14.3, 0.7)
  line L20 (-14.3, 0.7) -> (-14.3, 9.3)
  dimension "d123" = -0.3
  constraint coincident L2.end L3.start
  constraint coincident L0.start L15.end
extrude "Extrude12" cut sketch "Sketch1 (3)" against normal blind 6 draft -3 contours L0 L1 L2 L3 L15 L18 L19 L20 | L3 L15 L16 L17 L18 L20 | L0 L1 L2 L16 bodies 1 in component "base"
extrude "Extrude3'" cut sketch "Sketch1 (3)" against normal blind 6 draft -3 contours L0 L1 L2 L3 L15 L18 L19 L20 | L3 L15 L16 L17 L18 L20 | L0 L1 L2 L16 bodies 2 in component "lid"
sketch "Sketch2 (2)" plane through (0, 0, 10) normal (0, 0, 1) x (-1, 0, 0) in component "lid"
  line L0 (15, 16.9) -> (15, 19.9)
  line L1 (15, 19.9) -> (-15, 19.9)
  line L2 (-15, 19.9) -> (-15, 16.9)
  arc A0 (-17, 14.9) -> (-15, 16.9) centre (-17, 16.9) ccw
  line L3 (-17, 14.9) -> (-20, 14.9)
  line L4 (-20, 14.9) -> (-20, 8.5746)
  line L5 (-20, 8.5746) -> (-18.3387, 8.5746)
  arc A1 (-17.9789, 8) -> (-18.3387, 8.5746) centre (-18.3387, 8.1746) ccw
  line L6 (-17.9789, 8) -> (-19.0465, 5.8)
  arc A2 (-19.4063, 5.5746) -> (-19.0465, 5.8) centre (-19.4063, 5.9746) ccw
  line L7 (-19.4063, 5.5746) -> (-20, 5.5746)
  line L8 (-20, 5.5746) -> (-20, -14.9)
  line L9 (-20, -14.9) -> (-17, -14.9)
  arc A3 (-15, -16.9) -> (-17, -14.9) centre (-17, -16.9) ccw
  line L10 (-15, -16.9) -> (-15, -19.9)
  line L11 (-15, -19.9) -> (15, -19.9)
  line L12 (15, -19.9) -> (15, -16.9)
  arc A4 (17, -14.9) -> (15, -16.9) centre (17, -16.9) ccw
  line L13 (17, -14.9) -> (20, -14.9)
  line L14 (20, -14.9) -> (20, 14.9)
  line L15 (20, 14.9) -> (17, 14.9)
  arc A5 (15, 16.9) -> (17, 14.9) centre (17, 16.9) ccw
  circle A6 centre (-4.5, 0.1) radius 13.625
  point P0 (-4.5, 0.1)
  dimension "d128" = 27.25
  constraint coincident P0 A6.centre
  measures "d128" diameter of A6
extrude "Extrude4'" cut sketch "Sketch2 (2)" against normal through all contours A6 bodies 2 in component "lid"
fillet "Fillet1" radius 1.25 1 edges at (17.203, -5.027, 10) on bodies 2 in component "lid"
sketch "Sketch1 (4)" plane through (0, 0, 1) normal (0, 0, 1) x (-1, 0, 0) in component "driver and stator"
  line L0 (14, 14.1757) -> (-14, 14.1757)
  line L1 (-14, 14.1757) -> (-14, 10.4)
  arc A0 (-14, 10.4) -> (-19.5, -1.2082) centre (-4.5, -1.2082) ccw
  arc A1 (-19.5, -1.2082) -> (-1.4582, -19.25) centre (-1.4582, -1.2082) ccw
  arc A2 (-1.4582, -19.25) -> (19.5, 1.7082) centre (-1.4582, 1.7082) ccw
  arc A3 (19.5, 1.7082) -> (14.0854, 15.8058) centre (-1.5598, 1.7082) ccw
  line L2 (14.0854, 15.8058) -> (14, 14.1757)
  circle A4 centre (-4.5, 0.1) radius 7
  point P0 (-4.5, 0.1)
  dimension "d131" = 14
  constraint coincident P0 A4.centre
  measures "d131" diameter of A4
extrude "Extrude1''" add sketch "Sketch1 (4)" along normal blind 1 separate body contours A4 makes body 3 in component "driver and stator"
sketch "Sketch2 (3)" plane through (0, 0, 2) normal (0, 0, 1) x (-1, 0, 0) in component "driver and stator"
  circle A0 centre (-4.5, 0.1) radius 7
  circle A1 centre (-4.5, 0.1) radius 2
  circle A2 centre (-4.5, 0.1) radius 3.5
  circle A3 centre (-4.5, 0.1) radius 5.5
  circle A4 centre (-4.5, 0.1) radius 6.5
  line L0 (-4.5, 0.1) -> (-4.5, -6.4) construction
  line L1 (-6, -3.1863) -> (-6, -4.92)
  arc A5 (-6.2642, -5.1094) -> (-6, -4.92) centre (-6.2, -4.92) ccw
  arc A6 (-7.25, -4.6631) -> (-7.75, -5.5292) centre (-7.5, -5.0962) ccw
  line L2 (-7.75, -5.5292) -> (-7.25, -4.6631) construction
  arc A7 (-6, -3.1863) -> (-6.1081, -3.0087) centre (-6.2, -3.1863) ccw
  arc A8 (-2.8919, -3.0087) -> (-3, -3.1863) centre (-2.8, -3.1863) ccw
  line L3 (-3, -3.1863) -> (-3, -4.92)
  arc A9 (-3, -4.92) -> (-2.7358, -5.1094) centre (-2.8, -4.92) ccw
  arc A10 (-1.25, -5.5292) -> (-1.75, -4.6631) centre (-1.5, -5.0962) ccw
  line L4 (-6.7472, -4.92) -> (-2.2528, -4.92)
  arc A11 (-1.2137, -1.4) -> (-1.3913, -1.5081) centre (-1.2137, -1.6) ccw
  line L5 (-1.2137, -1.4) -> (0.52, -1.4)
  arc A12 (0.7094, -1.6642) -> (0.52, -1.4) centre (0.52, -1.6) ccw
  line L6 (0.52, -2.1472) -> (0.52, 2.3472)
  arc A13 (0.2631, -2.65) -> (1.1292, -3.15) centre (0.6962, -2.9) ccw
  arc A14 (1.1292, 3.35) -> (0.2631, 2.85) centre (0.6962, 3.1) ccw
  arc A15 (-1.3913, 1.7081) -> (-1.2137, 1.6) centre (-1.2137, 1.8) ccw
  arc A16 (0.52, 1.6) -> (0.7094, 1.8642) centre (0.52, 1.8) ccw
  line L7 (-1.2137, 1.6) -> (0.52, 1.6)
  arc A17 (-3, 3.3863) -> (-2.8919, 3.2087) centre (-2.8, 3.3863) ccw
  line L8 (-3, 3.3863) -> (-3, 5.12)
  arc A18 (-2.7358, 5.3094) -> (-3, 5.12) centre (-2.8, 5.12) ccw
  line L9 (-2.2528, 5.12) -> (-6.7472, 5.12)
  arc A19 (-1.75, 4.8631) -> (-1.25, 5.7292) centre (-1.5, 5.2962) ccw
  arc A20 (-7.75, 5.7292) -> (-7.25, 4.8631) centre (-7.5, 5.2962) ccw
  arc A21 (-6.1081, 3.2087) -> (-6, 3.3863) centre (-6.2, 3.3863) ccw
  arc A22 (-6, 5.12) -> (-6.2642, 5.3094) centre (-6.2, 5.12) ccw
  line L10 (-6, 3.3863) -> (-6, 5.12)
  arc A23 (-7.7863, 1.6) -> (-7.6087, 1.7081) centre (-7.7863, 1.8) ccw
  line L11 (-7.7863, 1.6) -> (-9.52, 1.6)
  arc A24 (-9.7094, 1.8642) -> (-9.52, 1.6) centre (-9.52, 1.8) ccw
  line L12 (-9.52, 2.3472) -> (-9.52, -2.1472)
  arc A25 (-9.2631, 2.85) -> (-10.1292, 3.35) centre (-9.6962, 3.1) ccw
  arc A26 (-10.1292, -3.15) -> (-9.2631, -2.65) centre (-9.6962, -2.9) ccw
  arc A27 (-7.6087, -1.5081) -> (-7.7863, -1.4) centre (-7.7863, -1.6) ccw
  arc A28 (-9.52, -1.4) -> (-9.7094, -1.6642) centre (-9.52, -1.6) ccw
  line L13 (-7.7863, -1.4) -> (-9.52, -1.4)
  circle A29 centre (-4.5, 0.1) radius 1.5
  circle A30 centre (-4.5, 0.1) radius 0.75
  circle A31 centre (-4.5, 0.1) radius 6
  dimension "d134" = 4
  dimension "d135" = 1.5
  dimension "d136" = 2
  dimension "d137" = 1
  dimension "d140" = 0.2
  dimension "d141" = 30
  dimension "d142" = 3
  dimension "d144" = 360
  dimension "d145" = 0.5
  dimension "d155" = 1.5
  constraint concentric A0 A1
  constraint concentric A1 A2
  constraint concentric A1 A3
  constraint concentric A3 A4
  constraint coincident A0.centre A1.centre
  constraint coincident A4 L0.end
  constraint vertical L0
  constraint parallel L0 L1
  constraint coincident A3 A5.start
  constraint tangent L1 A5
  constraint tangent A3 A5
  constraint coincident A3 A6.start
  constraint coincident A4 A6.end
  constraint coincident A6.centre L2
  constraint coincident A0.centre L2
  constraint coincident A2 A7.end
  constraint tangent L1 A7
  constraint tangent A2 A7
  constraint equal A5 A7
  constraint symmetric L0 L1.start A8.end
  constraint symmetric L0 L1.end L3.end
  constraint symmetric L0 A5.start A9.end
  constraint symmetric L0 A5 A9
  constraint symmetric L0 A6.end A10.start
  constraint symmetric L0 A6.start A10.end
  constraint symmetric L0 A6 A10
  constraint symmetric L0 A7.end A8.start
  constraint symmetric L0 A7 A8
  constraint coincident A3 L4.start
  constraint coincident A3 L4.end
  constraint horizontal L4
  constraint coincident A5.centre L4
  constraint concentric A3 A29
  constraint concentric A2 A30
  constraint concentric A30 A31
  constraint coincident A6.centre A31
  measures "d134" diameter of A1
  measures "d135" distance of A1 A2
  measures "d136" distance of A2 A3
  measures "d137" distance of A3 A4
  measures "d140" radius of A5
  measures "d141" angle of L0 L2
  measures "d142" distance of L1 L3
  measures "d145" distance of A1 A29
  measures "d155" diameter of A30
extrude "Extrude2''" add sketch "Sketch2 (3)" along normal blind 4 from surface at 1 separate body contours A1 makes body 4 in component "driver and stator"
extrude "Extrude3''" add sketch "Sketch2 (3)" along normal blind 2.5 from surface at 2 separate body contours A2 | A2 A11 L5 L6 A15 L7 | A2 A17 L8 L9 A21 L10 | A2 L1 A7 A8 L3 L4 | A3 A12 L6 A16 | A2 A23 L11 L12 A27 L13 | A3 A18 L9 A22 | A3 A13 A14 A31 | A3 A5 A9 L4 | A3 A19 A20 A31 | A3 A6 A10 A31 | A3 A24 L12 A28 | A4 A13 A14 A31 | A3 A25 A26 A31 | A4 A19 A20 A31 | A4 A6 A10 A31 | A4 A25 A26 A31 makes body 5 in component "driver and stator"
extrude "Extrude4''" add sketch "Sketch2 (3)" along normal blind 0.5 from surface at 4.5 separate body contours A2 | A2 A11 L5 L6 A15 L7 | A2 A17 L8 L9 A21 L10 | A2 L1 A7 A8 L3 L4 | A3 A12 L6 A16 | A3 L6 A16 | A3 A12 L6 | A2 A23 L11 L12 A27 L13 | A3 A18 L9 A22 | A3 A18 L9 | A3 A13 A14 A31 | A3 A9 L4 | A3 A5 A9 L4 | A3 L9 A22 | A3 A19 A20 A31 | A3 A5 L4 | A3 A6 A10 A31 | A3 A24 L12 A28 | A3 A24 L12 | A3 L12 A28 | A3 A25 A26 A31 makes body 6 in component "driver and stator"
extrude "Extrude5'" add sketch "Sketch2 (3)" against normal blind 2.5 from surface at 5 separate body contours A29 makes body 7 in component "driver and stator"
chamfer "Chamfer1" distance 0.1 angle 45 2 edges at (5.8985, -0.6424, 7) (6.3647, 0.6232, 7) on bodies 4 in component "driver and stator"
chamfer "Chamfer2" distance 0.25 angle 45 4 edges at (5.8985, -0.6424, 7) (5.1992, 0.1712, 7) (5.1992, 0.1712, 4.5) (5.8985, -0.6424, 4.5) on bodies 7 in component "driver and stator"
fillet "Fillet1'" radius 0.3 20 edges at (0.3469, -1.6, 7) (1.3176, -1.6292, 7) (2.0251, -2.5749, 7) (2.9708, -3.2824, 7) (3, -4.2531, 7) (3, 4.0531, 7) (2.9708, 3.0824, 7) (2.0251, 2.3749, 7) (1.3176, 1.4292, 7) (0.3469, 1.4, 7) (8.6531, 1.4, 7) (7.6824, 1.4292, 7) (6.9749, 2.3749, 7) (6.0292, 3.0824, 7) (6, 4.0531, 7) (6, -4.2531, 7) (6.0292, -3.2824, 7) (6.9749, -2.5749, 7) (7.6824, -1.6292, 7) (8.6531, -1.6, 7) on bodies 6 in component "driver and stator"
ref_plane "WorkPlane1" through (4.5, -0.1, 5.25) normal (0, 0, 1) x (-1, 0, 0) in component "driver and stator"
mirror "Mirror1" about plane through (4.5, -0.1, 5.25) normal (0, 0, 1) of bodies 6 makes body 8 in component "driver and stator"
sketch "Sketch3 (2)" plane through (0, 4.92, 0) normal (0, -1, 0) x (1, 0, 0) in component "driver and stator"
  arc A0 (6, 6.7) -> (5.7, 7) centre (5.7, 6.7) ccw
  line L0 (6, 6.7) -> (6, 6.5)
  line L1 (3, 6.5) -> (3, 6.7)
  arc A1 (3.3, 7) -> (3, 6.7) centre (3.3, 6.7) ccw
  arc A2 (3, 3.8) -> (3.3, 3.5) centre (3.3, 3.8) ccw
  line L2 (3, 3.8) -> (3, 4)
  line L3 (6, 4) -> (6, 3.8)
  arc A3 (5.7, 3.5) -> (6, 3.8) centre (5.7, 3.8) ccw
  line L4 (3.3, 7) -> (5.7, 7)
  line L5 (6, 6.5) -> (6, 4)
  line L6 (5.7, 3.5) -> (3.3, 3.5)
  line L7 (3, 4) -> (3, 6.5)
  arc A4 (5.7, 3) -> (6.5, 3.8) centre (5.7, 3.8) ccw
  line L8 (6.5, 4) -> (6.5, 3.8)
  line L9 (6.5, 6.5) -> (6.5, 4)
  line L10 (6.5, 6.7) -> (6.5, 6.5)
  arc A5 (6.5, 6.7) -> (5.7, 7.5) centre (5.7, 6.7) ccw
  line L11 (3.3, 7.5) -> (5.7, 7.5)
  arc A6 (3.3, 7.5) -> (2.5, 6.7) centre (3.3, 6.7) ccw
  line L12 (2.5, 6.5) -> (2.5, 6.7)
  line L13 (2.5, 4) -> (2.5, 6.5)
  line L14 (2.5, 3.8) -> (2.5, 4)
  arc A7 (2.5, 3.8) -> (3.3, 3) centre (3.3, 3.8) ccw
  line L15 (5.7, 3) -> (3.3, 3)
  dimension "d163" = -0.5
  constraint coincident A1.start L4.start
  constraint coincident A0.end L4.end
  constraint coincident L0.end L5.start
  constraint coincident L3.start L5.end
  constraint coincident A3.start L6.start
  constraint coincident A2.end L6.end
  constraint coincident L2.end L7.start
  constraint coincident L1.start L7.end
extrude "Extrude6'" add sketch "Sketch3 (2)" along normal up to surface (1.7336 mm away) separate body makes body 9 in component "driver and stator"
pattern_circular "C-Pattern1" count 4 over 360 about axis through (4.5, -0.1, 7) along (0, 0, -1) of bodies 9 makes body 10 at (9.52, -1.7667, 5.6667) makes body 11 at (2.8333, -5.12, 5.6667) makes body 12 at (-0.52, 1.5667, 5.6667) in component "driver and stator"
sketch "Sketch1 (5)" plane through (4.5, -0.1, 5.25) normal (0, 0, 1) x (1, 0, 0) in component "rotor"
  circle A0 centre (0, 0) radius 8
  circle A1 centre (0, 0) radius 7.75
  circle A2 centre (0, 0) radius 6.875
  line L0 (4.4192, 5.2666) -> (4.9816, 5.9368)
  line L1 (0, 0) -> (0, 6.4851) construction
  line L2 (-4.4192, 5.2666) -> (-4.9816, 5.9368)
  line L3 (-5.2666, 4.4192) -> (-5.9368, 4.9816)
  line L4 (-5.2666, -4.4192) -> (-5.9368, -4.9816)
  line L5 (-4.4192, -5.2666) -> (-4.9816, -5.9368)
  line L6 (4.4192, -5.2666) -> (4.9816, -5.9368)
  line L7 (5.2666, -4.4192) -> (5.9368, -4.9816)
  line L8 (5.2666, 4.4192) -> (5.9368, 4.9816)
  circle A3 centre (0, 0) radius 0.75
  dimension "d168" = 16
  dimension "d169" = 0.25
  dimension "d170" = 13.75
  dimension "d175" = 80
  dimension "d177" = 360
  dimension "d180" = 1.5
  constraint coincident A0.centre A1.centre
  constraint coincident A2 L0.start
  constraint coincident A1 L0.end
  constraint coincident A0.centre L0
  constraint vertical L1
  constraint symmetric L0.start L1 L2.start
  constraint symmetric L0.end L1 L2.end
  measures "d168" diameter of A0
  measures "d169" distance of A0 A1
  measures "d170" diameter of A2
  measures "d175" angle of L0 L2
  measures "d180" diameter of A3
extrude "Extrude1'''" add sketch "Sketch1 (5)" along normal mid plane 5 separate body contours A0 | A1 A2 L7 L8 | A1 A2 L0 L8 | A1 A2 L6 L7 | A1 A2 L0 L2 | A1 A2 L5 L6 | A1 A2 L2 L3 | A1 A2 L4 L5 | A1 A2 L3 L4 makes body 13 in component "rotor"
fillet "Fillet1''" radius 0.5 1 edges at (-2.9586, -2.9929, 7.75) on bodies 13 in component "rotor"
shell "Shell1'" thickness 0.25 removed faces 19 at (4.5, 7.5101, 2.75) at (10.6437, -3.1855, 6.9167) at (9.6799, -4.6205, 6.9167) at (8.4105, -5.7545, 6.9167) at (-0.6799, -4.6205, 6.0833) at (-0.9665, -4.2694, 6.9167) at (-0.6799, 4.4205, 6.9167) at (0.3306, 5.3665, 6.9167) at (9.0205, 5.0799, 6.9167) at (11.1897, 1.4855, 6.9167) at (10.6437, -3.1855, 3.5833) at (9.6799, -4.6205, 3.5833) at (8.4105, -5.7545, 3.5833) at (-0.6799, -4.6205, 4.4167) at (-0.9665, -4.2694, 3.5833) at (-0.6799, 4.4205, 3.5833) at (0.3306, 5.3665, 3.5833) at (9.0205, 5.0799, 3.5833) at (11.1897, 1.4855, 3.5833) on bodies 13 in component "rotor"
extrude "Extrude2'''" add sketch "Sketch1 (5)" along normal mid plane 4 separate body contours A1 A2 L7 L8 | A1 A2 L0 L2 | A1 A2 L5 L6 | A1 A2 L3 L4 makes body 14 at (6.9805, 7.2423, 5.9167) makes body 15 at (12.1161, 1.3345, 4.5833) makes body 16 at (-3.1161, 1.3345, 5.9167) makes body 17 at (8.9082, -6.4742, 5.9167) in component "rotor"
extrude "Extrude3'''" add sketch "Sketch1 (5)" along normal blind 3.75 and the other way blind 1.75 separate body contours A3 makes body 18 in component "rotor"
chamfer "Chamfer1'" distance 0.25 angle 45 2 edges at (3.8008, -0.3712, 9) (3.8008, 0.1712, 3.5) on bodies 18 in component "rotor"
ref_plane "WorkPlane1" through (0, 0, 1.5) normal (0, 0, 1) x (1, 0, 0) in component "fan"
sketch "Sketch1 (6)" plane through (0, 0, 1.5) normal (0, 0, 1) x (1, 0, 0) in component "fan"
  circle A0 centre (4.5, -0.1) radius 8
  circle A1 centre (4.5, -0.1) radius 8
  circle A2 centre (4.5, -0.1) radius 8.5
  circle A3 centre (4.5, -0.1) radius 10
  circle A4 centre (4.5, -0.1) radius 11.5
  dimension "d187" = 0.5
  dimension "d188" = 1.5
  dimension "d205" = 1.5
  constraint concentric A0 A2
  constraint concentric A2 A3
  constraint concentric A0 A4
  measures "d187" distance of A0 A2
  measures "d188" distance of A2 A3
  measures "d205" distance of A3 A4
extrude "Extrude1''''" add sketch "Sketch1 (6)" along normal blind 8.25 separate body contours A0 A1 | A2 makes body 19 in component "fan"
extrude "Extrude5''" add sketch "Sketch1 (6)" along normal blind 2.5 contours A3 bodies 19 in component "fan"
fillet "Fillet1'''" radius 1 1 edges at (-3.4248, -3.1737, 9.75) on bodies 19 in component "fan"
fillet "Fillet1'''" radius 0.25 2 edges at (-3.4248, -3.1737, 4) (-4.8233, -3.7162, 4) on bodies 19 in component "fan"
shell "Shell1''" thickness 0.5 removed faces 1 at (7.0527, -1.3293, 1.5) on bodies 19 in component "fan"
extrude "Extrude2''''" add sketch "Sketch1 (6)" along normal blind 1 contours A4 bodies 19 in component "fan"
sketch "Sketch2 (4)" plane through (0, 0, 9.25) normal (0, 0, -1) x (1, 0, 0) in component "fan"
  circle A0 centre (4.5, 0.1) radius 7.5
  circle A1 centre (4.5, 0.1) radius 0.75
  circle A2 centre (4.5, 0.1) radius 0.75
  circle A3 centre (4.5, 0.1) radius 2.75
  dimension "d195" = 2
  constraint concentric A1 A3
  measures "d195" distance of A2 A3
extrude "Extrude3''''" add sketch "Sketch2 (4)" along normal blind 1.5 contours A3 bodies 19 in component "fan"